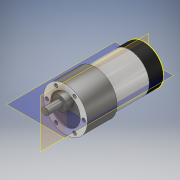
# Autodesk Inventor part: 251RPM-Motor
Saved by Autodesk Inventor 2018 (Build 220112000, 112)
## iProperties
Created: 2017-04-11
Part Number: 251RPM-Motor
Material: Generic
Document SubType Name: Modeling
Designer: jklei
Density: 1 g/cm^3
Appearance: Default
Author: jklei
Autodesk Inventor part; units mm, degrees
ref_plane "YZ Plane" through (0, 0, 0) normal (1, 0, 0) x (0, 1, 0)
ref_plane "XZ Plane" through (0, 0, 0) normal (0, 1, 0) x (-1, 0, 0)
ref_plane "XY Plane" through (0, 0, 0) normal (0, 0, 1) x (1, 0, 0)
sketch "Sketch1" plane through (0, 0, 0) normal (0, 0, 1) x (1, 0, 0)
  circle A0 centre (0, 0) radius 16.5
  dimension "d0" = 33
  constraints: 1 centre point, 1 coincident
  measures "d0" diameter of A0
extrude "Extrusion1" add sketch "Sketch1" along normal blind 29
sketch "Sketch2" plane through (0, 0, 29) normal (0, 0, 1) x (1, 0, 0)
  circle A0 centre (0, 0) radius 18.5
  dimension "d3" = 37
  constraints: 1 centre point, 1 coincident
  measures "d3" diameter of A0
extrude "Extrusion2" add sketch "Sketch2" along normal blind 24
sketch "Sketch3" plane through (0, 0, 53) normal (0, 0, 1) x (1, 0, 0)
  line L0 (0, 0) -> (0, 7)
  circle A0 centre (0, 7) radius 6
  dimension "d6" = 7
  dimension "d7" = 12
  constraints: 2 end point, 1 centre point, 1 coincident, 1 vertical
  measures "d6" distance of L0.start L0.end
  measures "d7" diameter of A0
extrude "Extrusion3" add sketch "Sketch3" along normal blind 6
sketch "Sketch4" plane through (0, 7, 59) normal (0, 0, 1) x (1, 0, 0)
  circle A0 centre (0, 0) radius 6 projected
  arc A1 (-1.199, 2.75) -> (1.199, 2.75) centre (0, 0) ccw
  line L0 (0, 0) -> (0, 2.75)
  line L1 (0, 2.75) -> (1.199, 2.75)
  line L2 (0, 2.75) -> (-1.199, 2.75)
  point P0 (0, -7)
  dimension "d10" = 6
  dimension "d11" = 2.75
  constraints: 6 end point, 2 horizontal, 2 point on circle, 1 centre point, 1 coincident, 1 vertical
  measures "d10" diameter of A1
  measures "d11" distance of L0.start L0.end
extrude "Extrusion4" add sketch "Sketch4" along normal blind 12 contours L2 L1 A1
sketch "Sketch5" plane through (0, 0, 0) normal (0, 0, -1) x (-1, 0, 0)
  circle A0 centre (0, 0) radius 16.45
  dimension "d16" = 32.9
  constraints: 1 centre point, 1 coincident
  measures "d16" diameter of A0
extrude "Extrusion5" add sketch "Sketch5" along normal blind 12
sketch "Sketch6" plane through (0, 0, 53) normal (0, 0, 1) x (1, 0, 0)
  circle A0 centre (0, 0) radius 18.5
  arc A1 (-3.1779, 12.0893) -> (3.1779, 12.0893) centre (0, 0) ccw
  circle A2 centre (0, 7) radius 6 projected
  dimension "d17" = 25
  constraints: 4 point on circle, 2 centre point, 2 coincident
  measures "d17" diameter of A1
extrude "Extrusion6" add sketch "Sketch6" along normal blind 1
sketch "Sketch8" plane through (0, 0, 54) normal (0, 0, 1) x (1, 0, 0)
  circle A0 centre (0, 0) radius 18.5 projected
  arc A1 (-3.1779, 12.0893) -> (3.1779, 12.0893) centre (0, 0) ccw projected
  line L0 (12.5, 0) -> (18.5, 0)
  circle A2 centre (15.5, 0) radius 1.5
  circle A3 centre (7.75, 13.4234) radius 1.5
  circle A4 centre (-7.75, 13.4234) radius 1.5
  circle A5 centre (-15.5, 0) radius 1.5
  circle A6 centre (-7.75, -13.4234) radius 1.5
  circle A7 centre (7.75, -13.4234) radius 1.5
  arc A8 (-1.199, 9.75) -> (1.199, 9.75) centre (0, 7) ccw projected
  line L1 (-1.199, 9.75) -> (1.199, 9.75) projected
  circle A9 centre (0, 7) radius 6 projected
  circle A10 centre (0, 7) radius 6 projected
  line L2 (1.199, 9.75) -> (-1.199, 9.75) projected
  arc A11 (-1.199, 9.75) -> (1.199, 9.75) centre (0, 7) ccw projected
  dimension "d44" = 3
  dimension "d47" = 360
  constraints: 6 centre point, 2 end point, 1 horizontal, 1 horizontal alignment, 1 midpoint, 1 point on circle, 14 other
  measures "d44" diameter of A2
extrude "Extrusion7" cut sketch "Sketch8" against normal blind 6 contours A2 L0 | L0 A2 | A3 | A4 | A5 | A6 | A7
thread "Thread7" size "5-40 UNC" class "2B" standard "ANSI Unified Screw Threads" full length
thread "Thread8" size "5-40 UNC" class "2B" standard "ANSI Unified Screw Threads" full length
thread "Thread9" size "5-40 UNC" class "2B" standard "ANSI Unified Screw Threads" full length
thread "Thread10" size "5-40 UNC" class "2B" standard "ANSI Unified Screw Threads" full length
thread "Thread11" size "5-40 UNC" class "2B" standard "ANSI Unified Screw Threads" full length
thread "Thread12" size "5-40 UNC" class "2B" standard "ANSI Unified Screw Threads" full length
sketch "Sketch9" plane through (0, 7, 71) normal (0, 0, 1) x (1, 0, 0)
  line L0 (1.199, 2.75) -> (-1.199, 2.75) projected
  arc A0 (-1.199, 2.75) -> (1.199, 2.75) centre (0, 0) ccw projected
  circle A1 centre (0, -7) radius 18.5 projected
  circle A2 centre (-7.75, -20.4234) radius 1.5 projected
  line L1 (0, 0) -> (-7.75, -20.4234)
  circle A3 centre (0, -7) radius 16.5 projected
  circle A4 centre (7.75, -20.4234) radius 1.5 projected
  circle A5 centre (-7.75, 6.4234) radius 1.5 projected
  line L2 (7.75, -20.4234) -> (-7.75, 6.4234)
  line L3 (0, -7) -> (-10.8253, -13.25)
  arc A6 (-3.1779, 5.0893) -> (3.1779, 5.0893) centre (0, -7) ccw projected
  line L4 (-16.8637, 0.607) -> (0, -7)
  line L5 (0, -7) -> (-16.8637, 0.607)
  line L6 (-16.8637, 0.607) -> (-26.1272, -19.9291)
  line L7 (-7.75, -20.4234) -> (-23.3448, -13.7609)
  line L8 (0, 0) -> (4.1821, 11.0211)
  line L9 (0, 0) -> (-13.8561, 5.2579)
  line L10 (-13.8561, 5.2579) -> (18.5, -7.0201)
  circle A7 centre (0, -7) radius 18.5 projected
  line L11 (0, 0) -> (18.5, -7.0201)
  constraints: 22 end point, 6 point on circle, 3 perpendicular, 2 collinear, 1 point on line, 2 other
sketch "Sketch10" plane through (0, 0, -12) normal (0, 0, -1) x (-1, 0, 0)
  circle A0 centre (0, 0) radius 16.5 projected
  line L0 (0, 16.5) -> (0, -16.5)
  line L1 (-16.5, 0) -> (16.5, 0)
  constraints: 4 end point, 4 point on circle, 1 perpendicular, 1 vertical
ref_plane "Work Plane1" through (16.5, 0, -12) normal (0, -1, 0) x (-1, 0, 0)
ref_plane "Work Plane2" through (0, 16.5, -12) normal (1, 0, 0) x (0, -1, 0)
body "Solid1"
